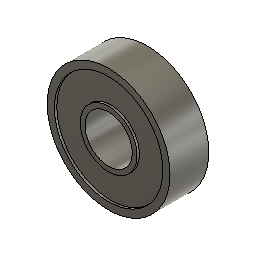
5mm ID Bearing (Autodesk Fusion 360 design; units mm, degrees)
Autodesk Fusion 360 part; units mm, degrees
sketch "Sketch1" plane through (0, 0, 12.7) normal (0, 0, 1) x (1, 0, 0)
  circle A0 centre (0, 0) radius 14.4875
  arc A1 (-50.5163, -35.9074) -> (-52.3626, -38.6593) centre (-31.1777, -50.8774) ccw
  arc A2 (-52.3626, -38.6593) -> (-51.5786, -39.6992) centre (0, 0) ccw
  arc A3 (-51.5786, -39.6992) -> (-48.4248, -38.6817) centre (-57.4938, -15.9697) ccw
  arc A4 (-47.7206, -38.8643) -> (-48.4248, -38.6817) centre (-48.197, -39.2522) ccw
  arc A5 (-47.7206, -38.8643) -> (-47.5821, -39.0337) centre (0, 0) ccw
  arc A6 (-47.5433, -39.7602) -> (-47.5821, -39.0337) centre (-48.0571, -39.4234) ccw
  arc A7 (-47.5433, -39.7602) -> (-49.168, -42.6485) centre (-27.0898, -53.1668) ccw
  arc A8 (-49.168, -42.6485) -> (-48.3048, -43.6237) centre (0, 0) ccw
  arc A9 (-48.3048, -43.6237) -> (-45.2406, -42.3618) centre (-56.0636, -20.4314) ccw
  arc A10 (-44.5242, -42.4886) -> (-45.2406, -42.3618) centre (-44.9687, -42.9127) ccw
  arc A11 (-44.5242, -42.4886) -> (-44.3729, -42.6466) centre (0, 0) ccw
  arc A12 (-44.2772, -43.3678) -> (-44.3729, -42.6466) centre (-44.8158, -43.0724) ccw
  arc A13 (-44.2772, -43.3678) -> (-45.6703, -46.3747) centre (-22.8349, -55.1283) ccw
  arc A14 (-45.6703, -46.3747) -> (-44.7333, -47.2791) centre (0, 0) ccw
  arc A15 (-44.7333, -47.2791) -> (-41.7775, -45.7808) centre (-54.2877, -24.7671) ccw
  arc A16 (-41.0534, -45.8509) -> (-41.7775, -45.7808) centre (-41.4632, -46.3086) ccw
  arc A17 (-41.0534, -45.8509) -> (-40.8901, -45.9966) centre (0, 0) ccw
  arc A18 (-40.7381, -46.7081) -> (-40.8901, -45.9966) centre (-41.2983, -46.4558) ccw
  arc A19 (-40.7381, -46.7081) -> (-41.891, -49.815) centre (-18.4392, -56.75) ccw
  arc A20 (-41.891, -49.815) -> (-40.8859, -50.6431) centre (0, 0) ccw
  arc A21 (-40.8859, -50.6431) -> (-38.0568, -48.9174) centre (-52.1772, -28.9501) ccw
  arc A22 (-37.3294, -48.9306) -> (-38.0568, -48.9174) centre (-37.702, -49.4191) ccw
  arc A23 (-37.3294, -48.9306) -> (-37.1552, -49.063) centre (0, 0) ccw
  arc A24 (-36.9478, -49.7604) -> (-37.1552, -49.063) centre (-37.5261, -49.5528) ccw
  arc A25 (-36.9478, -49.7604) -> (-37.8534, -52.9481) centre (-13.9298, -58.0218) ccw
  arc A26 (-37.8534, -52.9481) -> (-36.7864, -53.6949) centre (0, 0) ccw
  arc A27 (-36.7864, -53.6949) -> (-34.1014, -51.7526) centre (-49.7449, -32.9546) ccw
  arc A28 (-33.3753, -51.7086) -> (-34.1014, -51.7526) centre (-33.7084, -52.2248) ccw
  arc A29 (-33.3753, -51.7086) -> (-33.1912, -51.827) centre (0, 0) ccw
  arc A30 (-32.9298, -52.5058) -> (-33.1912, -51.827) centre (-33.5225, -52.3443) ccw
  arc A31 (-32.9298, -52.5058) -> (-33.5824, -55.7548) centre (-9.3345, -58.9358) ccw
  arc A32 (-33.5824, -55.7548) -> (-32.4602, -56.4156) centre (0, 0) ccw
  arc A33 (-32.4602, -56.4156) -> (-29.9358, -54.2686) centre (-47.006, -36.756) ccw
  arc A34 (-29.2154, -54.1678) -> (-29.9358, -54.2686) centre (-29.507, -54.7085) ccw
  arc A35 (-29.2154, -54.1678) -> (-29.0226, -54.2713) centre (0, 0) ccw
  arc A36 (-28.7087, -54.9276) -> (-29.0226, -54.2713) centre (-29.3123, -54.8131) ccw
  arc A37 (-28.7087, -54.9276) -> (-29.1044, -58.2178) centre (-4.6817, -59.4865) ccw
  arc A38 (-29.1044, -58.2178) -> (-27.9338, -58.7885) centre (0, 0) ccw
  arc A39 (-27.9338, -58.7885) -> (-25.5857, -56.45) centre (-43.9772, -40.3307) ccw
  arc A40 (-24.8754, -56.293) -> (-25.5857, -56.45) centre (-25.1237, -56.855) ccw
  arc A41 (-24.8754, -56.293) -> (-24.675, -56.3811) centre (0, 0) ccw
  arc A42 (-24.3106, -57.0108) -> (-24.675, -56.3811) centre (-24.9213, -56.9439) ccw
  arc A43 (-24.3106, -57.0108) -> (-24.447, -60.3219) centre (0, -59.6705) ccw
  arc A44 (-24.447, -60.3219) -> (-23.2352, -60.7989) centre (0, 0) ccw
  arc A45 (-23.2352, -60.7989) -> (-21.0778, -58.2834) centre (-40.6774, -43.6568) ccw
  arc A46 (-20.382, -58.0712) -> (-21.0778, -58.2834) centre (-20.5854, -58.6509) ccw
  arc A47 (-20.382, -58.0712) -> (-20.1754, -58.1433) centre (0, 0) ccw
  arc A48 (-19.7627, -58.7424) -> (-20.1754, -58.1433) centre (-20.3768, -58.7237) ccw
  arc A49 (-19.7627, -58.7424) -> (-19.6389, -62.054) centre (4.6817, -59.4865) ccw
  arc A50 (-19.6389, -62.054) -> (-18.3933, -62.4345) centre (0, 0) ccw
  arc A51 (-18.3933, -62.4345) -> (-16.44, -59.7575) centre (-37.1267, -46.7138) ccw
  arc A52 (-15.7629, -59.4913) -> (-16.44, -59.7575) centre (-15.9203, -60.0852) ccw
  arc A53 (-15.7629, -59.4913) -> (-15.5513, -59.547) centre (0, 0) ccw
  arc A54 (-15.0929, -60.1119) -> (-15.5513, -59.547) centre (-15.7065, -60.1414) ccw
  arc A55 (-15.0929, -60.1119) -> (-14.7096, -63.4035) centre (9.3345, -58.9358) ccw
  arc A56 (-14.7096, -63.4035) -> (-13.4381, -63.6852) centre (0, 0) ccw
  arc A57 (-13.4381, -63.6852) -> (-11.7008, -60.8632) centre (-33.3471, -49.4827) ccw
  arc A58 (-11.0467, -60.5447) -> (-11.7008, -60.8632) centre (-11.157, -61.1491) ccw
  arc A59 (-11.0467, -60.5447) -> (-10.8313, -60.5836) centre (0, 0) ccw
  arc A60 (-10.33, -61.1108) -> (-10.8313, -60.5836) centre (-10.9395, -61.1884) ccw
  arc A61 (-10.33, -61.1108) -> (-9.6897, -64.3622) centre (13.9298, -58.0218) ccw
  arc A62 (-9.6897, -64.3622) -> (-8.4, -64.5432) centre (0, 0) ccw
  arc A63 (-8.4, -64.5432) -> (-6.8894, -61.5936) centre (-29.362, -51.9465) ccw
  arc A64 (-6.2624, -61.2248) -> (-6.8894, -61.5936) centre (-6.3249, -61.8359) ccw
  arc A65 (-6.2624, -61.2248) -> (-6.0446, -61.2466) centre (0, 0) ccw
  arc A66 (-5.5035, -61.7329) -> (-6.0446, -61.2466) centre (-6.105, -61.858) ccw
  arc A67 (-5.5035, -61.7329) -> (-4.61, -64.924) centre (18.4392, -56.75) ccw
  arc A68 (-4.61, -64.924) -> (-3.3101, -65.0033) centre (0, 0) ccw
  arc A69 (-3.3101, -65.0033) -> (-2.0356, -61.9443) centre (-25.1958, -54.0901) ccw
  arc A70 (-1.4394, -61.5274) -> (-2.0356, -61.9443) centre (-1.4538, -62.1416) ccw
  arc A71 (-1.4394, -61.5274) -> (-1.2206, -61.5321) centre (0, 0) ccw
  arc A72 (-0.643, -61.9744) -> (-1.2206, -61.5321) centre (-1.2328, -62.1463) ccw
  arc A73 (-0.643, -61.9744) -> (0.4981, -65.0856) centre (22.8349, -55.1283) ccw
  arc A74 (0.4981, -65.0856) -> (1.8002, -65.0626) centre (0, 0) ccw
  arc A75 (1.8002, -65.0626) -> (2.8307, -61.913) centre (-20.8742, -55.9002) ccw
  arc A76 (3.3924, -61.4506) -> (2.8307, -61.913) centre (3.4263, -62.0641) ccw
  arc A77 (3.3924, -61.4506) -> (3.6109, -61.4382) centre (0, 0) ccw
  arc A78 (4.2214, -61.8338) -> (3.6109, -61.4382) centre (3.6469, -62.0515) ccw
  arc A79 (4.2214, -61.8338) -> (5.6031, -64.8459) centre (27.0898, -53.1668) ccw
  arc A80 (5.6031, -64.8459) -> (6.8994, -64.7208) centre (0, 0) ccw
  arc A81 (6.8994, -64.7208) -> (7.6797, -61.5001) centre (-16.424, -57.3657) ccw
  arc A82 (8.2033, -60.995) -> (7.6797, -61.5001) centre (8.2852, -61.6039) ccw
  arc A83 (8.2033, -60.995) -> (8.4201, -60.9655) centre (0, 0) ccw
  arc A84 (9.0598, -61.3119) -> (8.4201, -60.9655) centre (8.5042, -61.5741) ccw
  arc A85 (9.0598, -61.3119) -> (10.6736, -64.2064) centre (31.1777, -50.8774) ccw
  arc A86 (10.6736, -64.2064) -> (11.9561, -63.98) centre (0, 0) ccw
  arc A87 (11.9561, -63.98) -> (12.4812, -60.7079) centre (-11.8725, -58.4774) ccw
  arc A88 (12.9636, -60.1634) -> (12.4812, -60.7079) centre (13.093, -60.764) ccw
  arc A89 (12.9636, -60.1634) -> (13.1775, -60.1169) centre (0, 0) ccw
  arc A90 (13.8424, -60.4121) -> (13.1775, -60.1169) centre (13.309, -60.717) ccw
  arc A91 (13.8424, -60.4121) -> (15.6782, -63.171) centre (35.0734, -48.2744) ccw
  arc A92 (15.6782, -63.171) -> (16.939, -62.8447) centre (0, 0) ccw
  arc A93 (16.939, -62.8447) -> (17.2058, -59.5415) centre (-7.2478, -59.2287) ccw
  arc A94 (17.644, -58.9608) -> (17.2058, -59.5415) centre (17.8202, -59.5494) ccw
  arc A95 (17.644, -58.9608) -> (17.8536, -58.8977) centre (0, 0) ccw
  arc A96 (18.5396, -59.1398) -> (17.8536, -58.8977) centre (18.0318, -59.4856) ccw
  arc A97 (18.5396, -59.1398) -> (20.5863, -61.7462) centre (38.7529, -45.3738) ccw
  arc A98 (20.5863, -61.7462) -> (21.8176, -61.3219) centre (0, 0) ccw
  arc A99 (21.8176, -61.3219) -> (21.8244, -58.008) centre (-2.5785, -59.6147) ccw
  arc A100 (22.2156, -57.3947) -> (21.8244, -58.008) centre (22.4374, -57.9677) ccw
  arc A101 (22.2156, -57.3947) -> (22.4196, -57.3154) centre (0, 0) ccw
  arc A102 (23.1225, -57.5029) -> (22.4196, -57.3154) centre (22.6434, -57.8875) ccw
  arc A103 (23.1225, -57.5029) -> (25.3673, -59.9406) centre (42.1934, -42.1934) ccw
  arc A104 (25.3673, -59.9406) -> (26.5616, -59.4211) centre (0, 0) ccw
  arc A105 (26.5616, -59.4211) -> (26.3084, -56.1169) centre (2.1068, -59.6333) ccw
  arc A106 (26.6503, -55.4748) -> (26.3084, -56.1169) centre (26.9163, -56.0285) ccw
  arc A107 (26.6503, -55.4748) -> (26.8474, -55.3797) centre (0, 0) ccw
  arc A108 (27.5628, -55.5115) -> (26.8474, -55.3797) centre (27.1154, -55.9325) ccw
  arc A109 (27.5628, -55.5115) -> (29.992, -57.7656) centre (45.3738, -38.7529) ccw
  arc A110 (29.992, -57.7656) -> (31.1418, -57.1539) centre (0, 0) ccw
  arc A111 (31.1418, -57.1539) -> (30.6301, -53.8798) centre (6.7791, -59.2842) ccw
  arc A112 (30.9206, -53.2128) -> (30.6301, -53.8798) centre (31.2293, -53.744) ccw
  arc A113 (30.9206, -53.2128) -> (31.1097, -53.1025) centre (0, 0) ccw
  arc A114 (31.8332, -53.1778) -> (31.1097, -53.1025) centre (31.4202, -53.6326) ccw
  arc A115 (31.8332, -53.1778) -> (34.4318, -55.2343) centre (48.2744, -35.0734) ccw
  arc A116 (34.4318, -55.2343) -> (35.53, -54.5344) centre (0, 0) ccw
  arc A117 (35.53, -54.5344) -> (34.7631, -51.3105) centre (11.4096, -58.5695) ccw
  arc A118 (35.0004, -50.6228) -> (34.7631, -51.3105) centre (35.3497, -51.1281) ccw
  arc A119 (35.0004, -50.6228) -> (35.1801, -50.498) centre (0, 0) ccw
  arc A120 (35.9074, -50.5163) -> (35.1801, -50.498) centre (35.5313, -51.0021) ccw
  arc A121 (35.9074, -50.5163) -> (38.6593, -52.3626) centre (50.8774, -31.1777) ccw
  arc A122 (38.6593, -52.3626) -> (39.6992, -51.5786) centre (0, 0) ccw
  arc A123 (39.6992, -51.5786) -> (38.6817, -48.4248) centre (15.9697, -57.4938) ccw
  arc A124 (38.8643, -47.7206) -> (38.6817, -48.4248) centre (39.2522, -48.197) ccw
  arc A125 (38.8643, -47.7206) -> (39.0337, -47.5821) centre (0, 0) ccw
  arc A126 (39.7602, -47.5433) -> (39.0337, -47.5821) centre (39.4234, -48.0571) ccw
  arc A127 (39.7602, -47.5433) -> (42.6485, -49.168) centre (53.1668, -27.0898) ccw
  arc A128 (42.6485, -49.168) -> (43.6237, -48.3048) centre (0, 0) ccw
  arc A129 (43.6237, -48.3048) -> (42.3618, -45.2406) centre (20.4314, -56.0636) ccw
  arc A130 (42.4886, -44.5242) -> (42.3618, -45.2406) centre (42.9127, -44.9687) ccw
  arc A131 (42.4886, -44.5242) -> (42.6466, -44.3729) centre (0, 0) ccw
  arc A132 (43.3678, -44.2772) -> (42.6466, -44.3729) centre (43.0724, -44.8158) ccw
  arc A133 (43.3678, -44.2772) -> (46.3747, -45.6703) centre (55.1283, -22.8349) ccw
  arc A134 (46.3747, -45.6703) -> (47.2791, -44.7333) centre (0, 0) ccw
  arc A135 (47.2791, -44.7333) -> (45.7808, -41.7775) centre (24.7671, -54.2877) ccw
  arc A136 (45.8509, -41.0534) -> (45.7808, -41.7775) centre (46.3086, -41.4632) ccw
  arc A137 (45.8509, -41.0534) -> (45.9966, -40.8901) centre (0, 0) ccw
  arc A138 (46.7081, -40.7381) -> (45.9966, -40.8901) centre (46.4558, -41.2983) ccw
  arc A139 (46.7081, -40.7381) -> (49.815, -41.891) centre (56.75, -18.4392) ccw
  arc A140 (49.815, -41.891) -> (50.6431, -40.8859) centre (0, 0) ccw
  arc A141 (50.6431, -40.8859) -> (48.9174, -38.0568) centre (28.9501, -52.1772) ccw
  arc A142 (48.9306, -37.3294) -> (48.9174, -38.0568) centre (49.4191, -37.702) ccw
  arc A143 (48.9306, -37.3294) -> (49.063, -37.1552) centre (0, 0) ccw
  arc A144 (49.7604, -36.9478) -> (49.063, -37.1552) centre (49.5528, -37.5261) ccw
  arc A145 (49.7604, -36.9478) -> (52.9481, -37.8534) centre (58.0218, -13.9298) ccw
  arc A146 (52.9481, -37.8534) -> (53.6949, -36.7864) centre (0, 0) ccw
  arc A147 (53.6949, -36.7864) -> (51.7526, -34.1014) centre (32.9546, -49.7449) ccw
  arc A148 (51.7086, -33.3753) -> (51.7526, -34.1014) centre (52.2248, -33.7084) ccw
  arc A149 (51.7086, -33.3753) -> (51.827, -33.1912) centre (0, 0) ccw
  arc A150 (52.5058, -32.9298) -> (51.827, -33.1912) centre (52.3443, -33.5225) ccw
  arc A151 (52.5058, -32.9298) -> (55.7548, -33.5824) centre (58.9358, -9.3345) ccw
  arc A152 (55.7548, -33.5824) -> (56.4156, -32.4602) centre (0, 0) ccw
  arc A153 (56.4156, -32.4602) -> (54.2686, -29.9358) centre (36.756, -47.006) ccw
  arc A154 (54.1678, -29.2154) -> (54.2686, -29.9358) centre (54.7085, -29.507) ccw
  arc A155 (54.1678, -29.2154) -> (54.2713, -29.0226) centre (0, 0) ccw
  arc A156 (54.9276, -28.7087) -> (54.2713, -29.0226) centre (54.8131, -29.3123) ccw
  arc A157 (54.9276, -28.7087) -> (58.2178, -29.1044) centre (59.4865, -4.6817) ccw
  arc A158 (58.2178, -29.1044) -> (58.7885, -27.9338) centre (0, 0) ccw
  arc A159 (58.7885, -27.9338) -> (56.45, -25.5857) centre (40.3307, -43.9772) ccw
  arc A160 (56.293, -24.8754) -> (56.45, -25.5857) centre (56.855, -25.1237) ccw
  arc A161 (56.293, -24.8754) -> (56.3811, -24.675) centre (0, 0) ccw
  arc A162 (57.0108, -24.3106) -> (56.3811, -24.675) centre (56.9439, -24.9213) ccw
  arc A163 (57.0108, -24.3106) -> (60.3219, -24.447) centre (59.6705, 0) ccw
  arc A164 (60.3219, -24.447) -> (60.7989, -23.2352) centre (0, 0) ccw
  arc A165 (60.7989, -23.2352) -> (58.2834, -21.0778) centre (43.6568, -40.6774) ccw
  arc A166 (58.0712, -20.382) -> (58.2834, -21.0778) centre (58.6509, -20.5854) ccw
  arc A167 (58.0712, -20.382) -> (58.1433, -20.1754) centre (0, 0) ccw
  arc A168 (58.7424, -19.7627) -> (58.1433, -20.1754) centre (58.7237, -20.3768) ccw
  arc A169 (58.7424, -19.7627) -> (62.054, -19.6389) centre (59.4865, 4.6817) ccw
  arc A170 (62.054, -19.6389) -> (62.4345, -18.3933) centre (0, 0) ccw
  arc A171 (62.4345, -18.3933) -> (59.7575, -16.44) centre (46.7138, -37.1267) ccw
  arc A172 (59.4913, -15.7629) -> (59.7575, -16.44) centre (60.0852, -15.9203) ccw
  arc A173 (59.4913, -15.7629) -> (59.547, -15.5513) centre (0, 0) ccw
  arc A174 (60.1119, -15.0929) -> (59.547, -15.5513) centre (60.1414, -15.7065) ccw
  arc A175 (60.1119, -15.0929) -> (63.4035, -14.7096) centre (58.9358, 9.3345) ccw
  arc A176 (63.4035, -14.7096) -> (63.6852, -13.4381) centre (0, 0) ccw
  arc A177 (63.6852, -13.4381) -> (60.8632, -11.7008) centre (49.4827, -33.3471) ccw
  arc A178 (60.5447, -11.0467) -> (60.8632, -11.7008) centre (61.1491, -11.157) ccw
  arc A179 (60.5447, -11.0467) -> (60.5836, -10.8313) centre (0, 0) ccw
  arc A180 (61.1108, -10.33) -> (60.5836, -10.8313) centre (61.1884, -10.9395) ccw
  arc A181 (61.1108, -10.33) -> (64.3622, -9.6897) centre (58.0218, 13.9298) ccw
  arc A182 (64.3622, -9.6897) -> (64.5432, -8.4) centre (0, 0) ccw
  arc A183 (64.5432, -8.4) -> (61.5936, -6.8894) centre (51.9465, -29.362) ccw
  arc A184 (61.2248, -6.2624) -> (61.5936, -6.8894) centre (61.8359, -6.3249) ccw
  arc A185 (61.2248, -6.2624) -> (61.2466, -6.0446) centre (0, 0) ccw
  arc A186 (61.7329, -5.5035) -> (61.2466, -6.0446) centre (61.858, -6.105) ccw
  arc A187 (61.7329, -5.5035) -> (64.924, -4.61) centre (56.75, 18.4392) ccw
  arc A188 (64.924, -4.61) -> (65.0033, -3.3101) centre (0, 0) ccw
  arc A189 (65.0033, -3.3101) -> (61.9443, -2.0356) centre (54.0901, -25.1958) ccw
  arc A190 (61.5274, -1.4394) -> (61.9443, -2.0356) centre (62.1416, -1.4538) ccw
  arc A191 (61.5274, -1.4394) -> (61.5321, -1.2206) centre (0, 0) ccw
  arc A192 (61.9744, -0.643) -> (61.5321, -1.2206) centre (62.1463, -1.2328) ccw
  arc A193 (61.9744, -0.643) -> (65.0856, 0.4981) centre (55.1283, 22.8349) ccw
  arc A194 (65.0856, 0.4981) -> (65.0626, 1.8002) centre (0, 0) ccw
  arc A195 (65.0626, 1.8002) -> (61.913, 2.8307) centre (55.9002, -20.8742) ccw
  arc A196 (61.4506, 3.3924) -> (61.913, 2.8307) centre (62.0641, 3.4263) ccw
  arc A197 (61.4506, 3.3924) -> (61.4382, 3.6109) centre (0, 0) ccw
  arc A198 (61.8338, 4.2214) -> (61.4382, 3.6109) centre (62.0515, 3.6469) ccw
  arc A199 (61.8338, 4.2214) -> (64.8459, 5.6031) centre (53.1668, 27.0898) ccw
  arc A200 (64.8459, 5.6031) -> (64.7208, 6.8994) centre (0, 0) ccw
  arc A201 (64.7208, 6.8994) -> (61.5001, 7.6797) centre (57.3657, -16.424) ccw
  arc A202 (60.995, 8.2033) -> (61.5001, 7.6797) centre (61.6039, 8.2852) ccw
  arc A203 (60.995, 8.2033) -> (60.9655, 8.4201) centre (0, 0) ccw
  arc A204 (61.3119, 9.0598) -> (60.9655, 8.4201) centre (61.5741, 8.5042) ccw
  arc A205 (61.3119, 9.0598) -> (64.2064, 10.6736) centre (50.8774, 31.1777) ccw
  arc A206 (64.2064, 10.6736) -> (63.98, 11.9561) centre (0, 0) ccw
  arc A207 (63.98, 11.9561) -> (60.7079, 12.4812) centre (58.4774, -11.8725) ccw
  arc A208 (60.1634, 12.9636) -> (60.7079, 12.4812) centre (60.764, 13.093) ccw
  arc A209 (60.1634, 12.9636) -> (60.1169, 13.1775) centre (0, 0) ccw
  arc A210 (60.4121, 13.8424) -> (60.1169, 13.1775) centre (60.717, 13.309) ccw
  arc A211 (60.4121, 13.8424) -> (63.171, 15.6782) centre (48.2744, 35.0734) ccw
  arc A212 (63.171, 15.6782) -> (62.8447, 16.939) centre (0, 0) ccw
  arc A213 (62.8447, 16.939) -> (59.5415, 17.2058) centre (59.2287, -7.2478) ccw
  arc A214 (58.9608, 17.644) -> (59.5415, 17.2058) centre (59.5494, 17.8202) ccw
  arc A215 (58.9608, 17.644) -> (58.8977, 17.8536) centre (0, 0) ccw
  arc A216 (59.1398, 18.5396) -> (58.8977, 17.8536) centre (59.4856, 18.0318) ccw
  arc A217 (59.1398, 18.5396) -> (61.7462, 20.5863) centre (45.3738, 38.7529) ccw
  arc A218 (61.7462, 20.5863) -> (61.5371, 21.203) centre (0, 0) ccw
  circle A219 centre (-128.1176, 0) radius 6.6
  circle A220 centre (-128.1176, 0) radius 6.5
  circle A221 centre (-128.1176, 0) radius 2.5
  arc A222 (-54.5344, -35.53) -> (-51.3105, -34.7631) centre (-58.5695, -11.4096) ccw
  arc A223 (-50.6228, -35.0004) -> (-51.3105, -34.7631) centre (-51.1281, -35.3497) ccw
  arc A224 (-50.6228, -35.0004) -> (-50.498, -35.1801) centre (0, 0) ccw
  arc A225 (-50.5163, -35.9074) -> (-50.498, -35.1801) centre (-51.0021, -35.5313) ccw
  circle A226 centre (-128.1176, 0) radius 6.6
  line L0 (61.5371, 21.203) -> (61.5972, 21.2237)
  arc A227 (61.5972, 21.2237) -> (-25.8654, 59.7966) centre (0, 0) ccw
  line L1 (-25.8654, 59.7966) -> (-133.7898, 13.1133)
  arc A228 (-133.7898, 13.1133) -> (-131.9847, -13.7542) centre (-128.1176, 0) ccw
  line L2 (-131.9847, -13.7542) -> (-54.5344, -35.53)
  dimension "d65" = 13
  dimension "d66" = 5
  dimension "d75" = 0
  dimension "d76" = 0
  dimension "d77" = 0
  dimension "d78" = 0
  measures "d65" diameter of A220
  measures "d66" diameter of A221
extrude "Extrude1" add sketch "Sketch1" along normal blind 4.1 contours A220
sketch "Sketch2" plane through (0, 0, 16.8) normal (0, 0, 1) x (1, 0, 0)
  circle A0 centre (-128.1176, 0) radius 2.5
  circle A1 centre (-128.1176, 0) radius 6.5
  circle A2 centre (-128.1176, 0) radius 3.008
  circle A3 centre (-128.1176, 0) radius 5.738
  dimension "d69" = 0.508
  dimension "d70" = 0.762
extrude "Extrude2" cut sketch "Sketch2" against normal blind 0.254 contours A3
sketch "Sketch4" plane through (0, 0, 12.7) normal (0, 0, -1) x (-1, 0, 0)
  circle A0 centre (128.1176, 0) radius 2.5
  circle A1 centre (128.1176, 0) radius 6.5
  circle A2 centre (128.1176, 0) radius 3.008
  circle A3 centre (128.1176, 0) radius 5.738
extrude "Extrude3" cut sketch "Sketch4" against normal blind 0.254 contours A3
